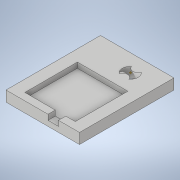
# Autodesk Inventor part: Part3
Saved by Autodesk Inventor 2021 (Build 250183000, 183)
## iProperties
Created: 2021-01-21
Part Number: Part3
Material: Generic
Document SubType Name: Modeling
Designer: kimsl
Density: 1 g/cm^3
Appearance: Default
Author: kimsl
Autodesk Inventor part; units mm, degrees
ref_plane "YZ Plane" through (0, 0, 0) normal (1, 0, 0) x (0, 1, 0)
ref_plane "XZ Plane" through (0, 0, 0) normal (0, 1, 0) x (-1, 0, 0)
ref_plane "XY Plane" through (0, 0, 0) normal (0, 0, 1) x (1, 0, 0)
sketch "Sketch1" plane through (0, 0, 0) normal (0, 1, 0) x (-1, 0, 0)
  line L0 (-34.98, 44.98) -> (34.98, 44.98)
  line L1 (34.98, 44.98) -> (34.98, -44.98)
  line L2 (34.98, -44.98) -> (-34.98, -44.98)
  line L3 (-34.98, -44.98) -> (-34.98, 44.98)
  line L4 (-34.98, 44.98) -> (34.98, -44.98) construction
  line L5 (34.98, 44.98) -> (-34.98, -44.98) construction
  point P0 (0, 0)
  dimension "d0" = 89.96
  dimension "d1" = 69.96
  constraints: 12 end point, 2 midpoint, 2 parallel, 1 horizontal, 1 perpendicular
  measures "d0" distance of L0.end L1.end
  measures "d1" distance of L1.end L2.end
extrude "Extrusion1" add sketch "Sketch1" along normal blind 10
sketch "Sketch2" plane through (0, 10, 0) normal (0, 1, 0) x (1, 0, 0)
  circle A0 centre (10, 28.2843) radius 7.52
  line L0 (-34.98, 44.98) -> (-34.98, -44.98) projected
  point P0 (0, 0)
  dimension "d4" = 30
  dimension "d5" = 15.04
  dimension "d6" = 44.98
  constraints: 1 centre point
  measures "d4" distance of point (0, 0) A0.centre
  measures "d5" diameter of A0
  measures "d6" distance from line of L0 A0.centre
sketch "Sketch3" plane through (0, 10, 0) normal (0, 1, 0) x (1, 0, 0)
  line L0 (24.02, -38.04) -> (-24.02, -38.04)
  line L1 (-24.02, -38.04) -> (-24.02, 12)
  line L2 (-24.02, 12) -> (24.02, 12)
  line L3 (24.02, 12) -> (24.02, -38.04)
  line L4 (24.02, -38.04) -> (-24.02, 12) construction
  line L5 (-24.02, -38.04) -> (24.02, 12) construction
  point P0 (0, 0)
  point P1 (0, -13.02)
  dimension "d9" = 12
  dimension "d10" = 50.04
  dimension "d11" = 48.04
  dimension "d12" = 0
  constraints: 12 end point, 2 midpoint, 2 parallel, 1 horizontal, 1 perpendicular
  measures "d9" distance from line of point (0, 0) L2
  measures "d10" distance between parallel lines of L2 L0
  measures "d11" distance between parallel lines of L3 L1
  measures "d12" horizontal distance of point (0, 0) point (0, -13.02)
extrude "Extrusion3" cut sketch "Sketch3" against normal blind 5.04
extrude "Extrusion4" cut sketch "Sketch2" against normal through all
sketch "Sketch6" plane through (-34.98, 0, 44.98) normal (0, 0, 1) x (1, 0, 0)
  line L0 (39.98, 5) -> (49.98, 5)
  line L1 (49.98, 5) -> (49.98, 15)
  line L2 (49.98, 15) -> (39.98, 15)
  line L3 (39.98, 15) -> (39.98, 5)
  line L4 (37.46, 10) -> (52.5, 10) projected
  line L5 (39.98, 5) -> (49.98, 15) construction
  line L6 (49.98, 5) -> (39.98, 15) construction
  point P0 (34.98, 0)
  point P1 (44.98, 10)
  dimension "d29" = 10
  dimension "d30" = 10
  constraints: 12 end point, 3 midpoint, 2 parallel, 1 horizontal, 1 perpendicular
  measures "d29" distance of L0.end L1.end
  measures "d30" distance of L1.end L2.end
extrude "Extrusion5" cut sketch "Sketch6" against normal blind 33
sketch "Sketch7" plane through (0, 10, 0) normal (0, 1, 0) x (1, 0, 0)
  circle A0 centre (10, 28.2843) radius 7.52 projected
  circle A1 centre (10, 35.8043) radius 5
  circle A2 centre (10, 20.7643) radius 5
  point P0 (0, 0)
  dimension "d34" = 10
  dimension "d35" = 10
  dimension "d36" = 15.04
  constraints: 2 centre point, 2 point on circle, 1 vertical alignment
  measures "d34" diameter of A1
  measures "d35" diameter of A2
  measures "d36" distance of A1.centre A2.centre
coil "Coil2" sketch "Sketch7" operation add axis through (0, -10, 0) along (0, -1, 0) pitch 50 turns 0.2 hand left contours A2 A0 | A0 A2
sketch "Sketch8" plane through (0, 10, 0) normal (0, 1, 0) x (1, 0, 0)
  arc A0 (14.7156, 22.4265) -> (5.2844, 22.4265) centre (10, 28.2843) ccw projected
  circle A1 centre (10, 35.8043) radius 5
  point P0 (0, 0)
  point P1 (10, 35.8043)
  dimension "d45" = 10
  constraints: 3 point on circle, 1 centre point, 1 coincident
  measures "d45" diameter of A1
coil "Coil3" sketch "Sketch8" operation add axis through (0, -10, 0) along (0, -1, 0) pitch 50 turns 0.2 hand right
sketch "Sketch9" plane through (34.98, 0, -44.98) normal (1, 0, 0) x (0, 0, -1)
  line L0 (-89.96, 10) -> (0, 10) projected
  line L1 (0, 0) -> (-38.9181, 0) projected
  line L2 (-89.96, 10) -> (0, 10)
  line L3 (0, 10) -> (0, 0)
  line L4 (0, 0) -> (-89.96, 0)
  line L5 (-89.96, 0) -> (-89.96, 10)
  point P0 (-44.98, 0)
  constraints: 8 end point, 2 parallel, 1 horizontal, 1 perpendicular
extrude "Extrusion6" cut sketch "Sketch9" along normal blind 20
body "Solid1"
